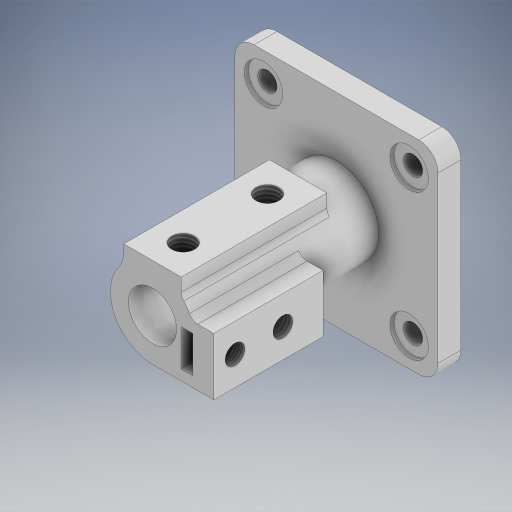
# Autodesk Inventor part: A1.3
Saved by Autodesk Inventor 2024 (Build 280153000, 153)
## iProperties
Created: 2024-01-30
Part Number: A1.3
Material: Generic
Document SubType Name: Modeling
Designer: Alex
Density: 1 g/cm^3
Appearance: Default
Author: Alex
Autodesk Inventor part; units mm, degrees
sketch "Sketch1" plane through (0, 0, 0) normal (0, 0, 1) x (1, 0, 0)
  line L0 (-53, -53) -> (53, -53)
  line L1 (53, -53) -> (53, 53)
  line L2 (53, 53) -> (-53, 53)
  line L3 (-53, 53) -> (-53, -53)
  line L4 (-53, -53) -> (53, 53) construction
  line L5 (53, -53) -> (-53, 53) construction
  line L6 (38, 38) -> (38, -38) construction
  line L7 (38, -38) -> (-38, -38) construction
  line L8 (-38, -38) -> (-38, 38) construction
  line L9 (-38, 38) -> (38, 38) construction
  circle A0 centre (38, 38) radius 5
  circle A1 centre (-38, 38) radius 5
  circle A2 centre (38, -38) radius 5
  circle A3 centre (-38, -38) radius 5
  circle A4 centre (-38, 38) radius 10
  circle A5 centre (38, 38) radius 10
  circle A6 centre (38, -38) radius 10
  circle A7 centre (-38, -38) radius 10
  point P0 (0, 0)
  dimension "d0" = 106
  dimension "d1" = 106
  dimension "d2" = 15
  dimension "d3" = 10
  dimension "d4" = 10
  dimension "d5" = 10
  dimension "d6" = 10
  dimension "d7" = 20
  dimension "d8" = 20
  dimension "d9" = 20
  dimension "d10" = 20
  constraints: 20 end point, 8 centre point, 8 coincident, 4 parallel, 2 midpoint, 2 perpendicular, 1 horizontal, 3 other
  measures "d0" distance of L2.end L1.end
  measures "d1" distance of L1.end L0.end
  measures "d2" distance between parallel lines of L1 L6
  measures "d3" diameter of A0
  measures "d4" diameter of A1
  measures "d5" diameter of A2
  measures "d6" diameter of A3
  measures "d7" diameter of A4
  measures "d8" diameter of A5
  measures "d9" diameter of A6
  measures "d10" diameter of A7
extrude "Extrusion1" add sketch "Sketch1" against normal blind 12 contours L3 L2 L1 L0 | A4 | A5 | A6 | A7
extrude "Extrusion2" cut sketch "Sketch1" against normal blind 2 contours A4 | A5 | A6 | A7
sketch "Sketch2" plane through (0, 0, 0) normal (0, 0, 1) x (1, 0, 0)
  circle A0 centre (0, 0) radius 22
  dimension "d15" = 44
  constraints: 1 centre point, 1 coincident
  measures "d15" diameter of A0
extrude "Extrusion3" add sketch "Sketch2" along normal blind 96
sketch "Sketch3" plane through (0, 0, 96) normal (0, 0, 1) x (1, 0, 0)
  circle A0 centre (0, 0) radius 22 construction
  constraints: 1 centre point, 1 coincident
hole "Hole1" at (0, 0, 96) direction (0, 0, -1) diameter 25 depth 82 tip angle 118
ref_plane "Work Plane2" through (0, 25, 0) normal (0, 1, 0) x (-1, 0, 0)
sketch "Sketch7" plane through (0, 25, 0) normal (0, 1, 0) x (-1, 0, 0)
  line L0 (22, 96) -> (-22, 96) construction
  line L1 (-22, 0) -> (22, 0) construction
  line L2 (15, 96) -> (-15, 96)
  line L3 (-15, 96) -> (-15, 20)
  line L4 (-15, 20) -> (15, 20)
  line L5 (15, 20) -> (15, 96)
  line L6 (15, 96) -> (-15, 20) construction
  line L7 (-15, 96) -> (15, 20) construction
  line L8 (22, 0) -> (22, 96) construction
  line L9 (-22, 0) -> (-22, 96) construction
  point P0 (0, 0)
  point P1 (0, 58)
  dimension "d33" = 30
  dimension "d34" = 76
  dimension "d35" = 7
  constraints: 12 end point, 2 midpoint, 2 parallel, 1 collinear, 1 horizontal, 1 perpendicular
  measures "d33" distance of L4.end L3.end
  measures "d34" distance of L3.end L2.end
  measures "d35" distance between parallel lines of L8 L5
extrude "Extrusion6" add sketch "Sketch7" against normal up to next
ref_plane "Work Plane3" through (32, 0, 0) normal (1, 0, 0) x (0, 1, 0)
sketch "Sketch8" plane through (32, 0, 0) normal (1, 0, 0) x (0, 1, 0)
  line L0 (16.0935, 96) -> (-22, 96) construction
  line L1 (-22, 0) -> (-22, 96) construction
  line L2 (22, 0) -> (22, 20) construction
  line L3 (-53, 0) -> (53, 0) construction
  line L4 (-22, 96) -> (8, 96)
  line L5 (8, 96) -> (8, 39)
  line L6 (8, 39) -> (-22, 39)
  line L7 (-22, 39) -> (-22, 96)
  point P0 (0, 0)
  dimension "d39" = 30
  dimension "d40" = 57
  constraints: 8 end point, 2 parallel, 1 horizontal, 1 perpendicular
  measures "d39" distance of L5.end L6.end
  measures "d40" distance of L4.end L5.end
extrude "Extrusion7" add sketch "Sketch8" against normal up to next
ref_plane "Work Plane4" through (21, 0, 0) normal (1, 0, 0) x (0, 0, -1)
sketch "Sketch10" plane through (0, 25, 0) normal (0, 1, 0) x (1, 0, 0)
  line L0 (15, -96) -> (15, -20) construction
  line L1 (15, -20) -> (-15, -20) construction
  line L2 (-15, -20) -> (-15, -96) construction
  line L3 (-15, -96) -> (15, -96) construction
  line L4 (-15, -96) -> (15, -96) construction
  line L5 (15, -96) -> (15, -80) construction
  line L6 (15, -80) -> (-15, -80) construction
  line L7 (-15, -80) -> (-15, -96) construction
  line L8 (-15, -80) -> (15, -80) construction
  line L9 (15, -80) -> (15, -36) construction
  line L10 (15, -36) -> (-15, -36) construction
  line L11 (-15, -36) -> (-15, -80) construction
  line L12 (0, -20) -> (0, -96) construction
  circle A0 centre (0, -36) radius 6
  circle A1 centre (0, -80) radius 6
  point P0 (0, 0)
  dimension "d49" = 16
  dimension "d50" = 44
  dimension "d51" = 12
  dimension "d52" = 12
  constraints: 18 end point, 4 midpoint, 4 parallel, 4 point on line, 2 centre point, 2 horizontal, 2 perpendicular
  measures "d49" distance of L5.end L4.end
  measures "d50" distance of L9.end L8.end
  measures "d51" diameter of A0
  measures "d52" diameter of A1
extrude "Extrusion9" cut sketch "Sketch10" against normal up to surface
thread "Thread1" size "M14x2" class "6H" standard "ANSI Metric M Profile" full length
thread "Thread2" size "M14x2" class "6H" standard "ANSI Metric M Profile" full length
sketch "Sketch11" plane through (32, 0, 0) normal (1, 0, 0) x (0, 0, -1)
  line L0 (-39, -22) -> (-39, 8) construction
  line L1 (-39, 8) -> (-96, 8) construction
  line L2 (-96, 8) -> (-96, -22) construction
  line L3 (-96, -22) -> (-39, -22) construction
  line L4 (-96, -7) -> (-39, -7) construction
  line L5 (-96, -22) -> (-39, -22) construction
  line L6 (-96, -22) -> (-85, -22) construction
  line L7 (-85, -22) -> (-85, 8) construction
  line L8 (-85, 8) -> (-96, 8) construction
  line L9 (-96, 8) -> (-96, -22) construction
  line L10 (-85, -22) -> (-60, -22) construction
  line L11 (-60, -22) -> (-60, 8) construction
  line L12 (-60, 8) -> (-85, 8) construction
  line L13 (-85, 8) -> (-85, -22) construction
  circle A0 centre (-85, -7) radius 5.1
  circle A1 centre (-60, -7) radius 5.1
  point P0 (0, 0)
  dimension "d59" = 11
  dimension "d60" = 25
  dimension "d61" = 10.2
  dimension "d62" = 10.2
  constraints: 18 end point, 4 midpoint, 4 parallel, 2 centre point, 2 horizontal, 2 perpendicular, 2 point on line
  measures "d59" distance of L8.end L7.end
  measures "d60" distance of L12.end L11.end
  measures "d61" diameter of A0
  measures "d62" diameter of A1
extrude "Extrusion10" cut sketch "Sketch11" against normal blind 11
thread "Thread3" size "M12x1.75" class "6H" standard "ANSI Metric M Profile" length 11
thread "Thread4" size "M11x1.5" class "6H" standard "ANSI Metric M Profile" length 11
fillet "Fillet1" radius 5 2 edges at (20.4939, 8, 67.5) (15, 16.0935, 58)
fillet "Fillet2" radius 15 1 edges at (-15, 16.0935, 58)
fillet "Fillet3" radius 10 4 edges at (-53, 53, -6) (53, 53, -6) (-53, -53, -6) (53, -53, -6)
sketch "Sketch12" plane through (0, 0, 96) normal (0, 0, 1) x (1, 0, 0)
  line L0 (15, 2.5) -> (21, 2.5)
  line L1 (21, 2.5) -> (21, -16.5)
  line L2 (21, -16.5) -> (15, -16.5)
  line L3 (15, -16.5) -> (15, 2.5)
  circle A0 centre (0, 0) radius 12.5 construction
  arc A1 (19.282, 10.5926) -> (16.2963, 14.7794) centre (0, 0) ccw construction
  arc A2 (15, 18.1384) -> (16.2963, 14.7794) centre (20, 18.1384) ccw construction
  line L4 (15, 25) -> (15, 18.1384) construction
  line L5 (-15, 25) -> (15, 25) construction
  line L6 (-15, 25) -> (-15, 21.6564) construction
  arc A3 (-17.8378, 12.8768) -> (-15, 21.6564) centre (-30, 21.6564) ccw construction
  arc A4 (-17.8378, 12.8768) -> (0, -22) centre (0, 0) ccw construction
  line L7 (32, -22) -> (0, -22) construction
  line L8 (32, 8) -> (32, -22) construction
  line L9 (32, 8) -> (23.6643, 8) construction
  arc A5 (19.282, 10.5926) -> (23.6643, 8) centre (23.6643, 13) ccw construction
  line L10 (32, -7) -> (-20.8567, -7) construction
  point P0 (21, -7)
  dimension "d72" = 6
  dimension "d73" = 19
  dimension "d74" = 11
  constraints: 10 end point, 2 horizontal, 2 midpoint, 2 parallel, 1 perpendicular, 1 point on circle, 1 point on line
  measures "d72" distance of L1.end L2.end
  measures "d73" distance of L0.end L1.end
  measures "d74" distance between parallel lines of L8 L1
extrude "Extrusion11" cut sketch "Sketch12" against normal blind 48
body "Solid1"
